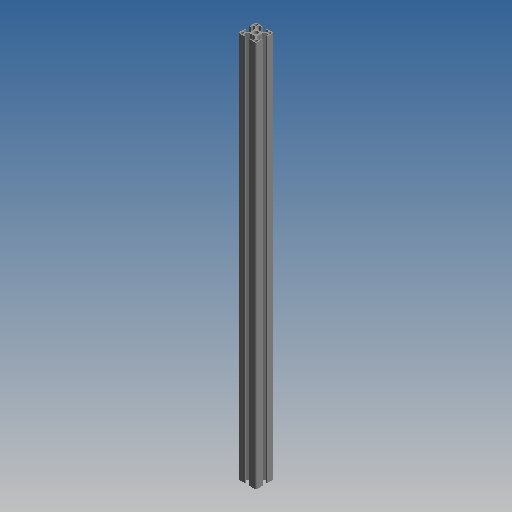
# Autodesk Inventor part: HFS6-3030-650
Saved by Autodesk Inventor 2020 (Build 240168000, 168)
## iProperties
Part Number: HFS6-3030-650
Material: 一般
Catalog Web Link: www.cadenas.de
Description: NEFS6-3030, NEFSB6-3030, EFS6-3030, EFSB6-3030, HFS6-3030, HFSB6-3030, CAF6-3030, HFSY6-3030, NFSL6-3030,  HFSL6-3030, HFSLB6-3030, GFS6-3030-HFS6 Series Aluminum Extrusions 30 Square -1 Slot-
Vendor: MISUMI
Document SubType Name: Modeling
Designer: partserver
Manufacturer: MISUMI
Mass: 215.744 g
Surface Area: 2048.8 cm^2
Volume: 215.744 cm^3
Density: 1 g/cm^3
Appearance: PSOLRGB-175-175-175
Category: PARTsolutions
Company: MISUMI
PSOL_IDENT_0: {$CADENAS_DATA\23d-libs\misumi\metric\38_al_extrusions_blackets\6\hfs6_3030.prj},720 {VTYP=3D},{NB=H
PSOL_IDENT_1: FS6-3030-650},{LINA=HFS6-3030-650},{NN=NEFS6-3030, NEFSB6-3030, EFS6-3030, EFSB6-3030, HFS6-3030, HF
PSOL_IDENT_2: SB6-3030, CAF6-3030, HFSY6-3030, NFSL6-3030,  HFSL6-3030, HFSLB6-3030, GFS6-3030},{DATE=30.10.2020 1
PSOL_IDENT_3: 6:28:01},{GEOMDATE=08.06.2016 01:16:00},{VERSION=},{LINEID=130},{WBVAR=L,ALT1,ALT2,ALT3,ALT4,ALT5,CP
PSOL_IDENT_4: 5,DL5,DR5,ALT6,ALT9,ALT10,ALT11,DD6SE,DD6,HP6,NHL6,DL6,NHR6,DR6,ALT7,ALT8,NH9,AH,BH,CH,DH,EH,NH10,AV
PSOL_IDENT_5: ,BV,CV,DV,EV,NH11,AP,BP,CP,DP,EP,ALT12,ALT13,Z,NH12,XA,XB,XC,XD,XE,NH13,YA,YB,YC,YD,YE,ALT14,HP14,DL
PSOL_IDENT_6: 14,DR14,ALT15,HP15,DL15,DR15,ALT16,HP16,DL16,DR16,ALT17,HQ17,JLP,ALT19,ALT20},{WBNUMERIC=L,DD6,NH9,A
PSOL_IDENT_7: H,BH,CH,DH,EH,NH10,AV,BV,CV,DV,EV,NH11,AP,BP,CP,DP,EP,NH12,XA,XB,XC,XD,XE,NH13,YA,YB,YC,YD,YE,HQ17,J
PSOL_IDENT_8: LP}  {NB=HFS6-3030-650},{LINA=HFS6-3030-650},{KT=DUMMY},{PN=HFS6-3030-650},{TPS=HFS6-3030},{MAT=A6N0
PSOL_IDENT_9: 1SS-T5 Aluminum Alloy},{ST=Clear Anodize},{FRMW=30},{FRMH=30},{FRD=6.8},{L=650.0},{MASS=0.90},{SA=33
PSOL_IDENT_10: 3},{LX=2.83x10^4},{LY=2.83x10^4},{ALT1=},{M1=0},{IDM1=6.647},{DALT1=4.2},{DPL1=0},{DPR1=0},{ALT1PN=}
PSOL_IDENT_11: ,{ALT2=},{ALT2ALG= '','w/o End Tapping (Heli-Coil Insert)','LHP','with LHP (Tapping on the Left (Hel
PSOL_IDENT_12: i-Coil Insert))','RHP','with RHP (Tapping on the Right (Heli-Coil Insert))','HPW','with HPW (Tapping
PSOL_IDENT_13: on Both Ends (Heli-Coil Insert))' },{M2=0},{DP2=0},{ALT2PN=},{ALT3=},{ALT3ALG= '','w/o Tapping (Cor
PSOL_IDENT_14: ner Section)','LSP','with LSP (Tapping (Corner Section))','RSP','with RSP (Tapping (Corner Section))'
PSOL_IDENT_15: ,'SPW','with SPW (Tapping (Corner Section))' },{M3=0},{IDM3=4.134},{DP3=0},{ALT3PN=},{ALT4=},{ALT4AL
PSOL_IDENT_16: G= '', 'w/o SC (High Precision Cut)', 'SC', 'with SC (High Precision Cut)' },{ALT4PN=},{ALT5=},{ALT5
PSOL_IDENT_17: ALG= '','w/o 45 Degree Cut','1','with 45 Degree Cut' },{CP5=},{CP5ALG= '','N/A' },{DL5=},{DL5ALG= ''
PSOL_IDENT_18: ,'N/A' },{DR5=},{DR5ALG= '','N/A' },{FRMLALT5=0},{FRMRALT5=0},{ALT5PN=},{ALT6=},{ALT6ALG= '','w/o Fa
PSOL_IDENT_19: stening Location Wrench Access Hole Alterations','1','with Fastening Location Wrench Access Hole Alt
PSOL_IDENT_20: erations' },{ALT9=},{ALT9ALG= '','w/o Location Specified Wrench Access Hole Alteratons (Horizontal)'
PSOL_IDENT_21: ,'1','with Location Specified Wrench Access Hole Alteratons (Horizontal)' },{ALT10=},{ALT10ALG= '','
PSOL_IDENT_22: w/o Location Specified Wrench Access Hole Alteratons (Vertical)','1','with Location Specified Wrench
PSOL_IDENT_23: Access Hole Alteratons (Vertical)' },{ALT11=},{ALT11ALG= '','w/o Location Specified Wrench Access H
PSOL_IDENT_24: ole Alteratons (Crisscross)','1','with Location Specified Wrench Access Hole Alteratons (Crisscross)'
PSOL_IDENT_25: },{DD6SE=},{DD6SEALG= '','N/A' },{DD6=0},{DD6ALG=0},{HP6=},{HP6ALG= '','N/A' },{NHL6=},{NHL6ALG= ''
PSOL_IDENT_26: ,'N/A' },{DL6=},{DL6ALG= '','N/A' },{NHR6=},{NHR6ALG= '','N/A' },{DR6=},{DR6ALG= '','N/A' },{DD6PN=}
PSOL_IDENT_27: ,{HL6=0},{HL6D=0},{HR6=0},{HR6D=0},{J6=0},{J6D=0},{K6=0},{K6D=0},{ALT7=},{ALT7ALG= '','N/A' },{ALT8=
PSOL_IDENT_28: },{ALT8ALG= '','N/A' },{ALT678PN=},{NH9=0},{NH9MAX=5},{NH9ALG=[0]},{AH=0.0},{AHMIN=7},{AHMAX=645},{A
PSOL_IDENT_29: HALG=[0]},{BH=0.0},{BHMIN=2},{BHMAX=647},{BHALG=[0]},{CH=0.0},{CHMIN=2},{CHMAX=649},{CHALG=[0]},{DH=
PSOL_IDENT_30: 0.0},{DHMIN=2},{DHMAX=651},{DHALG=[0]},{EH=0.0},{EHMIN=2},{EHMAX=643},{EHALG=[0]},{NH10=0},{NH10MAX=
PSOL_IDENT_31: 5},{NH10ALG=[0]},{AV=0.0},{AVMIN=7},{AVMAX=645},{AVALG=[0]},{BV=0.0},{BVMIN=2},{BVMAX=647},{BVALG=[0
PSOL_IDENT_32: ]},{CV=0.0},{CVMIN=2},{CVMAX=649},{CVALG=[0]},{DV=0.0},{DVMIN=2},{DVMAX=651},{DVALG=[0]},{EV=0.0},{E
PSOL_IDENT_33: VMIN=2},{EVMAX=643},{EVALG=[0]},{NH11=0},{NH11MAX=5},{NH11ALG=[0]},{AP=0.0},{APMIN=7},{APMAX=645},{A
PSOL_IDENT_34: PALG=[0]},{BP=0.0},{BPMIN=2},{BPMAX=647},{BPALG=[0]},{CP=0.0},{CPMIN=2},{CPMAX=649},{CPALG=[0]},{DP=
PSOL_IDENT_35: 0.0},{DPMIN=2},{DPMAX=651},{DPALG=[0]},{EP=0.0},{EPMIN=2},{EPMAX=643},{EPALG=[0]},{ALT9PN=},{ALT10PN=
PSOL_IDENT_36: },{ALT11PN=},{ALT91011PN=},{ALT12=},{ALT12ALG= '','w/o Counterbore Hole in Specified Position (Verti
PSOL_IDENT_37: cal)','1','with Counterbore Hole in Specified Position (Vertical)' },{ALT13=},{ALT13ALG= '','w/o Cou
PSOL_IDENT_38: nterbore Hole in Specified Position (Horizontal)','1','with Counterbore Hole in Specified Position (
PSOL_IDENT_39: Horizontal)' },{Z=},{ZALG= '','N/A' },{DD12=0.0},{DD112=0.0},{NH12=0},{NH12MAX=5},{NH12ALG=[0]},{XA=
PSOL_IDENT_40: 0.0},{XAMIN=7},{XAMAX=645},{XAALG=[0]},{XB=0.0},{XBMIN=2},{XBMAX=647},{XBALG=[0]},{XC=0.0},{XCMIN=2}
PSOL_IDENT_41: ,{XCMAX=649},{XCALG=[0]},{XD=0.0},{XDMIN=2},{XDMAX=651},{XDALG=[0]},{XE=0.0},{XEMIN=2},{XEMAX=643},{
PSOL_IDENT_42: XEALG=[0]},{NH13=0},{NH13MAX=5},{NH13ALG=[0]},{YA=0.0},{YAMIN=7},{YAMAX=645},{YAALG=[0]},{YB=0.0},{Y
PSOL_IDENT_43: BMIN=2},{YBMAX=647},{YBALG=[0]},{YC=0.0},{YCMIN=2},{YCMAX=649},{YCALG=[0]},{YD=0.0},{YDMIN=2},{YDMAX=
PSOL_IDENT_44: 651},{YDALG=[0]},{YE=0.0},{YEMIN=2},{YEMAX=643},{YEALG=[0]},{ALT12PN=},{ALT13PN=},{ALT1213PN=},{ALT1
PSOL_IDENT_45: 4=},{ALT14ALG= '','w/o D Type Hole Alteration','1','with D Type Hole Alteration' },{HP14=},{HP14ALG=
PSOL_IDENT_46: '','N/A' },{DL14=},{DL14ALG= '','N/A' },{DR14=},{DR14ALG= '','N/A' },{H14=0},{D14=0.0},{ALT14PN=},{
PSOL_IDENT_47: ALT15=},{ALT15ALG= '','w/o S Type Hole Alteration','1','with S Type Hole Alteration' },{HP15=},{HP15
PSOL_IDENT_48: ALG= '','N/A' },{DL15=},{DL15ALG= '','N/A' },{DR15=},{DR15ALG= '','N/A' },{H15=0},{D115=0.0},{D215=0
PSOL_IDENT_49: .0},{ALT15PN=},{ALT16=},{ALT16ALG= '','w/o M Type Hole Alteration','1','with M Type Hole Alteration'
PSOL_IDENT_50: },{HP16=},{HP16ALG= '','N/A' },{DL16=},{DL16ALG= '','N/A' },{DR16=},{DR16ALG= '','N/A' },{H116=0},{
PSOL_IDENT_51: D16=0.0},{ALT16PN=},{ALT17=},{ALT17ALG= '','w/o L Type Hole Alteration (Top)','1','with L Type Hole
PSOL_IDENT_52: Alteration (Top)' },{HQ17=0},{HQ17ALG=0},{JLP=0},{JLPMIN=4.9},{JLPMAX=0},{JLPALG=[0]},{L17=0},{D17=0
PSOL_IDENT_53: .0},{ALT17PN=},{ALT19=},{ALT19ALG= '','N/A' },{M19=0},{DP19=0},{ALT19PN=},{ALT20=},{ALT20PN=},{ERROR
PSOL_IDENT_54: ALT01=OK},{ERRORALT02=OK},{ERRORALT03=OK},{ERRORALT05=OK},{ERRORALT06091=OK},{ERRORALT06092=OK},{ERR
PSOL_IDENT_55: ORALT06093=OK},{ERRORALT06094=OK},{ERRORALT06101=OK},{ERRORALT06102=OK},{ERRORALT06103=OK},{ERRORALT
PSOL_IDENT_56: 06104=OK},{ERRORALT06111=OK},{ERRORALT06112=OK},{ERRORALT06113=OK},{ERRORALT06114=OK},{ERRORALT06121=
PSOL_IDENT_57: OK},{ERRORALT06122=OK},{ERRORALT06123=OK},{ERRORALT06124=OK},{ERRORALT06131=OK},{ERRORALT06132=OK},{
PSOL_IDENT_58: ERRORALT06133=OK},{ERRORALT06134=OK},{ERRORALT0614=OK},{ERRORALT0615=OK},{ERRORALT0616=OK},{ERRORALT
PSOL_IDENT_59: 06171=OK},{ERRORALT06172=OK},{ERRORALT06173=OK},{ERRORALT0619=OK},{ERRORALT0911=OK},{ERRORALT0913=OK
PSOL_IDENT_60: },{ERRORALT0914=OK},{ERRORALT0915=OK},{ERRORALT0916=OK},{ERRORALT0917=OK},{ERRORALT0919=OK},{ERRORAL
PSOL_IDENT_61: T1011=OK},{ERRORALT1012=OK},{ERRORALT1014=OK},{ERRORALT1015=OK},{ERRORALT1016=OK},{ERRORALT1017=OK},
PSOL_IDENT_62: {ERRORALT1019=OK},{ERRORALT1112=OK},{ERRORALT1113=OK},{ERRORALT1114=OK},{ERRORALT1115=OK},{ERRORALT1
PSOL_IDENT_63: 116=OK},{ERRORALT1117=OK},{ERRORALT1119=OK},{ERRORALT1214=OK},{ERRORALT1215=OK},{ERRORALT1216=OK},{E
PSOL_IDENT_64: RRORALT1217=OK},{ERRORALT1219=OK},{ERRORALT1314=OK},{ERRORALT1315=OK},{ERRORALT1316=OK},{ERRORALT131
PSOL_IDENT_65: 7=OK},{ERRORALT1319=OK},{ERRORALT1415=OK},{ERRORALT1416=OK},{ERRORALT1417=OK},{ERRORALT1419=OK},{ERR
PSOL_IDENT_66: ORALT1516=OK},{ERRORALT1517=OK},{ERRORALT1519=OK},{ERRORALT1617=OK},{ERRORALT1619=OK},{ERRORALT1719=
PSOL_IDENT_67: OK},{ERRORPN=}
NB: HFS6-3030-650
NN: NEFS6-3030, NEFSB6-3030, EFS6-3030, EFSB6-3030, HFS6-3030, HFSB6-3030, CAF6-3030, HFSY6-3030, NFSL6-3030,  HFSL6-3030, HFSLB6-3030, GFS6-3030
NT: HFS6 Series Aluminum Extrusions 30 Square -1 Slot-
NBSYN: $PN.
LINA: HFS6-3030-650
CATALOG: Misumi
PN: HFS6-3030-650
TPS: HFS6-3030
MAT: A6N01SS-T5 Aluminum Alloy
ST: Clear Anodize
L: 650
MASS: 0.90
SA: 333
LX: 2.83x10^4
LY: 2.83x10^4
ALT1: w/o End Tapping
M1: 0
DPL1: 0
DPR1: 0
ALT2: w/o End Tapping (Heli-Coil Insert)
M2: 0
DP2: 0
ALT3: w/o Tapping (Corner Section)
M3: 0
DP3: 0
ALT4: w/o SC (High Precision Cut)
ALT5: w/o 45 Degree Cut
CP5: N/A
DL5: N/A
DR5: N/A
ALT6: w/o Fastening Location Wrench Access Hole Alterations
ALT9: w/o Location Specified Wrench Access Hole Alteratons (Horizontal)
ALT10: w/o Location Specified Wrench Access Hole Alteratons (Vertical)
ALT11: w/o Location Specified Wrench Access Hole Alteratons (Crisscross)
DD6SE: N/A
DD6: 0
HP6: N/A
NHL6: N/A
DL6: N/A
NHR6: N/A
DR6: N/A
HL6D: 0
HR6D: 0
J6D: 0
K6D: 0
ALT7: N/A
ALT8: N/A
NH9: 0
AH: 0
BH: 0
CH: 0
DH: 0
EH: 0
NH10: 0
AV: 0
BV: 0
CV: 0
DV: 0
EV: 0
NH11: 0
AP: 0
BP: 0
CP: 0
DP: 0
EP: 0
ALT12: w/o Counterbore Hole in Specified Position (Vertical)
ALT13: w/o Counterbore Hole in Specified Position (Horizontal)
Z: N/A
DD12: 0
DD112: 0
NH12: 0
XA: 0
XB: 0
XC: 0
XD: 0
XE: 0
NH13: 0
YA: 0
YB: 0
YC: 0
YD: 0
YE: 0
ALT14: w/o D Type Hole Alteration
HP14: N/A
DL14: N/A
DR14: N/A
H14: 0
D14: 0
ALT15: w/o S Type Hole Alteration
HP15: N/A
DL15: N/A
DR15: N/A
H15: 0
D115: 0
D215: 0
ALT16: w/o M Type Hole Alteration
HP16: N/A
DL16: N/A
DR16: N/A
H116: 0
D16: 0
ALT17: w/o L Type Hole Alteration (Top)
HQ17: 0
JLP: 0
D17: 0
ALT19: N/A
M19: 0
DP19: 0
ALT20: w/o CW (End Face C Chamfering)
SUPPLIER: MISUMI
ARTICLENO: HFS6-3030-650
BOMINFO: HFS6-3030-650
CREATOR: CADENAS GmbH
Title: HFS6-3030-650
Author: Cadenas PARTsolutions
Comments: HFS6 Series Aluminum Extrusions 30 Square -1 Slot-
Autodesk Inventor part; units mm, degrees
sketch "Sketch_1" plane through (0, 0, 0) normal (0, 0, 1) x (1, 0, 0)
  line L0 (-15, -4) -> (-15, -13)
  arc A0 (-15, -13) -> (-13, -15) centre (-13, -13) ccw
  line L1 (-13, -15) -> (-4, -15)
  line L2 (-4, -15) -> (-4, -13)
  line L3 (-4, -13) -> (-8.25, -13)
  line L4 (-8.25, -13) -> (-8.25, -9.6642)
  line L5 (-8.25, -9.6642) -> (-4.5858, -6)
  line L6 (-4.5858, -6) -> (-0.5196, -6)
  line L7 (-0.5196, -6) -> (0, -5.7)
  line L8 (0, -5.7) -> (0.5196, -6)
  line L9 (0.5196, -6) -> (4.5858, -6)
  line L10 (4.5858, -6) -> (8.25, -9.6642)
  line L11 (8.25, -9.6642) -> (8.25, -13)
  line L12 (8.25, -13) -> (4, -13)
  line L13 (4, -13) -> (4, -15)
  line L14 (4, -15) -> (13, -15)
  arc A1 (13, -15) -> (15, -13) centre (13, -13) ccw
  line L15 (15, -13) -> (15, -4)
  line L16 (15, -4) -> (13, -4)
  line L17 (13, -4) -> (13, -8.25)
  line L18 (13, -8.25) -> (9.6642, -8.25)
  line L19 (9.6642, -8.25) -> (6, -4.5858)
  line L20 (6, -4.5858) -> (6, -0.5196)
  line L21 (6, -0.5196) -> (5.7, 0)
  line L22 (5.7, 0) -> (6, 0.5196)
  line L23 (6, 0.5196) -> (6, 4.5858)
  line L24 (6, 4.5858) -> (9.6642, 8.25)
  line L25 (9.6642, 8.25) -> (13, 8.25)
  line L26 (13, 8.25) -> (13, 4)
  line L27 (13, 4) -> (15, 4)
  line L28 (15, 4) -> (15, 13)
  arc A2 (15, 13) -> (13, 15) centre (13, 13) ccw
  line L29 (13, 15) -> (4, 15)
  line L30 (4, 15) -> (4, 13)
  line L31 (4, 13) -> (8.25, 13)
  line L32 (8.25, 13) -> (8.25, 9.6642)
  line L33 (8.25, 9.6642) -> (4.5858, 6)
  line L34 (4.5858, 6) -> (0.5196, 6)
  line L35 (0.5196, 6) -> (0, 5.7)
  line L36 (0, 5.7) -> (-0.5196, 6)
  line L37 (-0.5196, 6) -> (-4.5858, 6)
  line L38 (-4.5858, 6) -> (-8.25, 9.6642)
  line L39 (-8.25, 9.6642) -> (-8.25, 13)
  line L40 (-8.25, 13) -> (-4, 13)
  line L41 (-4, 13) -> (-4, 15)
  line L42 (-4, 15) -> (-13, 15)
  arc A3 (-13, 15) -> (-15, 13) centre (-13, 13) ccw
  line L43 (-15, 13) -> (-15, 4)
  line L44 (-15, 4) -> (-13, 4)
  line L45 (-13, 4) -> (-13, 8.25)
  line L46 (-13, 8.25) -> (-9.6642, 8.25)
  line L47 (-9.6642, 8.25) -> (-6, 4.5858)
  line L48 (-6, 4.5858) -> (-6, 0.5196)
  line L49 (-6, 0.5196) -> (-5.7, 0)
  line L50 (-5.7, 0) -> (-6, -0.5196)
  line L51 (-6, -0.5196) -> (-6, -4.5858)
  line L52 (-6, -4.5858) -> (-9.6642, -8.25)
  line L53 (-9.6642, -8.25) -> (-13, -8.25)
  line L54 (-13, -8.25) -> (-13, -4)
  line L55 (-13, -4) -> (-15, -4)
  constraints: 112 end point, 8 point on circle, 4 centre point
extrude "Extrusion1" add sketch "Sketch_1" against normal blind 650
sketch "Sketch2" plane through (0, 0, -650) normal (0, 0, -1) x (-1, 0, 0)
  point P0 (0, 0)
hole "Hole1" at (0, 0, -650) direction (0, 0, 1) diameter 6.8 depth 650
sketch "Sketch3" plane through (0, 0, -650) normal (0, 0, -1) x (-1, 0, 0)
  point P0 (-11.6, 11.6)
hole "Hole2" at (11.6, 11.6, -650) direction (0, 0, 1) diameter 4.2 depth 650
pattern_linear "Rectangular Pattern1" count 2 spacing 23.2 along (-1, 0, 0) count 2 spacing 23.2 along (0, -1, 0) of "Hole2"
ref_plane "C1_XY" through (0, 0, 0) normal (0, 0, 1) x (1, 0, 0)
ref_plane "C1_YZ" through (0, 0, 0) normal (1, 0, 0) x (0, 1, 0)
ref_plane "C1_ZX" through (0, 0, 0) normal (0, 1, 0) x (0, 0, 1)
ref_plane "to_frame_cap1_XY" through (0, 0, 0) normal (0, 0, 1) x (1, 0, 0)
ref_plane "to_frame_cap1_YZ" through (0, 0, 0) normal (1, 0, 0) x (0, 1, 0)
ref_plane "to_frame_cap1_ZX" through (0, 0, 0) normal (0, 1, 0) x (0, 0, 1)
ref_plane "to_frame_cap2_XY" through (0, 0, -650) normal (0, 0, -1) x (1, 0, 0)
ref_plane "to_frame_cap2_YZ" through (0, 0, -650) normal (1, 0, 0) x (0, -1, 0)
ref_plane "to_frame_cap2_ZX" through (0, 0, -650) normal (0, -1, 0) x (0, 0, -1)
body "Solid1"
